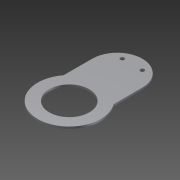
# Autodesk Inventor part: JointC3'cover2_2nd
Saved by Autodesk Inventor 2011 (Build 150239000, 239)
## iProperties
Created: 2013-02-08
Part Number: JointC3'cover2_2nd
Document SubType Name: Modeling
Designer: JohnHenry
Density: 1 g/cm^3
Author: JohnHenry
Autodesk Inventor part; units mm, degrees
ref_plane "YZ Plane" through (0, 0, 0) normal (1, 0, 0) x (0, 1, 0)
ref_plane "XZ Plane" through (0, 0, 0) normal (0, 1, 0) x (-1, 0, 0)
ref_plane "XY Plane" through (0, 0, 0) normal (0, 0, 1) x (1, 0, 0)
sketch "スケッチ1" plane through (0, 0, 0) normal (0, 0, 1) x (1, 0, 0)
  circle A0 centre (0, 0) radius 12.5
  circle A1 centre (-0.0318, -23.9) radius 15.75
  line L0 (-12.5, 0) -> (-12.5, -14.2768)
  line L1 (12.5, 0) -> (12.5, -14.3597)
  line L2 (-0.0318, 12.5) -> (-0.0318, -39.65)
  point P0 (-15.7818, -23.9)
  dimension "d0" = 25
  dimension "d1" = 31.5
  dimension "d2" = 23.9
  constraints: 6 end point, 6 point on circle, 2 centre point, 2 tangent, 1 coincident, 1 parallel, 1 vertical
  measures "d0" diameter of A0
  measures "d1" diameter of A1
  measures "d2" distance of A1.centre A0.centre
extrude "押し出し2" add sketch "スケッチ1" along normal blind 1
sketch "スケッチ4" plane through (0, 0, 0) normal (0, 0, -1) x (-1, 0, 0)
  arc A0 (12.5, 0) -> (-12.5, 0) centre (0, 0) ccw projected
  point P0 (-5, 7.5)
  point P1 (5, 7.5)
  dimension "d29" = 10
  dimension "d30" = 5
  dimension "d31" = 7.5
  dimension "d32" = 7.5
  measures "d29" distance of point (5, 7.5) point (-5, 7.5)
  measures "d30" horizontal distance of point (5, 7.5) A0.centre
  measures "d31" vertical distance of A0.centre point (5, 7.5)
  measures "d32" vertical distance of A0.centre point (-5, 7.5)
hole "Hole3" at (5, 7.5, 0) at (-5, 7.5, 0) direction (0, 0, 1) diameter 2 depth 8 tip angle 118
sketch "スケッチ5" plane through (0, 0, 0) normal (0, 0, -1) x (-1, 0, 0)
  arc A0 (-12.5, -14.3597) -> (12.5, -14.2768) centre (0.0318, -23.9) ccw projected
  constraints: 1 coincident
hole "Hole4" at (-0.0318, -23.9, 0) direction (0, 0, 1) diameter 20 end through all
equation "\"d32\" = d31"
